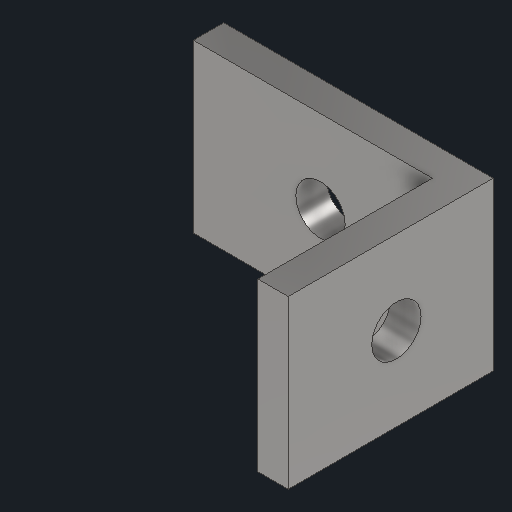
# Autodesk Inventor part: short_L_bracket
Saved by Autodesk Inventor 2025.2 (Build 292293000, 293)
## iProperties
Created: 2025-02-19
Part Number: short_L_bracket
Material: Stainless Steel
Document SubType Name: Modeling
Designer: turbo
Density: 8 g/cm^3
Appearance: Semi-Polished
Author: turbo
Autodesk Inventor part; units mm, degrees
ref_plane "YZ Plane" through (0, 0, 0) normal (1, 0, 0) x (0, 1, 0)
ref_plane "XZ Plane" through (0, 0, 0) normal (0, 1, 0) x (-1, 0, 0)
ref_plane "XY Plane" through (0, 0, 0) normal (0, 0, 1) x (1, 0, 0)
sketch "Sketch1" plane through (0, 0, 0) normal (0, 0, 1) x (1, 0, 0)
  circle A0 centre (0, -0.0008) radius 3.25 projected
  line L0 (-17, -11.2508) -> (-17, 11.2492) projected
  line L1 (19, -11.2508) -> (-17, -11.2508) projected
  line L2 (19, 11.2492) -> (19, -11.2508) projected
  line L3 (-17, 11.2492) -> (19, 11.2492) projected
  line L4 (18.75, -11.0008) -> (-16.75, -11.0008)
  line L5 (-16.75, -11.0008) -> (-16.75, 10.9992)
  line L6 (-16.75, 10.9992) -> (18.75, 10.9992)
  line L7 (18.75, 10.9992) -> (18.75, -11.0008)
  point P0 (0, 0)
  dimension "d0" = 0.25
  constraints: 8 end point, 3 other
  measures "d0" distance between parallel lines of L2 L7
extrude "Extrusion1" add sketch "Sketch1" along normal blind 4 contours L4 L5 L6 L7
sketch "Sketch2" plane through (18.75, -11.0008, 0) normal (1, 0, 0) x (0, 0, -1)
  circle A0 centre (-12.75, 11) radius 3.25 projected
  line L0 (-27.75, 22.25) -> (-27.75, 16.6789) projected
  line L1 (-4, 22) -> (-27, 22)
  line L2 (-27, 22) -> (-27, 0)
  line L3 (-27, 0) -> (-4, 0)
  line L4 (-4, 0) -> (-4, 22)
  line L5 (0, 0) -> (-4, 0) projected
  point P0 (0, 11.0008)
  dimension "d3" = 23
  constraints: 8 end point, 2 parallel, 1 collinear, 1 horizontal, 1 perpendicular
  measures "d3" distance of L3.end L2.end
extrude "Extrusion2" add sketch "Sketch2" against normal blind 4
body "Solid1"
